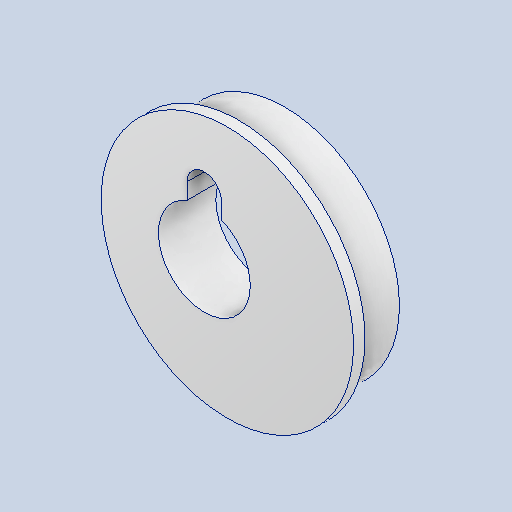
# Autodesk Inventor part: 偏心軸板
Saved by Autodesk Inventor 2024 (Build 280153000, 153)
## iProperties
Created: 2023-05-29
Part Number: 偏心軸板
Material: アルミニウム 6061
Document SubType Name: Modeling
Designer: yuta2
Density: 2.7 g/cm^3
Appearance: アルミニウム - フラット
Author: yuta2
Autodesk Inventor part; units mm, degrees
ref_plane "YZ Plane" through (0, 0, 0) normal (1, 0, 0) x (0, 1, 0)
ref_plane "XZ Plane" through (0, 0, 0) normal (0, 1, 0) x (-1, 0, 0)
ref_plane "XY Plane" through (0, 0, 0) normal (0, 0, 1) x (1, 0, 0)
sketch "スケッチ1" plane through (0, 0, 0) normal (0, 0, 1) x (1, 0, 0)
  circle A0 centre (0, 0) radius 10
  dimension "d0" = 20
  constraints: 1 centre point, 1 coincident
  measures "d0" diameter of A0
extrude "押し出し1" add sketch "スケッチ1" along normal blind 5
sketch "スケッチ2" plane through (0, 0, 5) normal (0, 0, 1) x (1, 0, 0)
  circle A0 centre (0, 0) radius 10 projected
  circle A1 centre (0, 0) radius 11
  circle A2 centre (0, 0) radius 10 projected
  dimension "d3" = 22
  constraints: 1 centre point, 1 coincident
  measures "d3" diameter of A1
extrude "押し出し2" add sketch "スケッチ2" against normal blind 1
sketch "スケッチ3" plane through (0, 0, 0) normal (0, 0, -1) x (-1, 0, 0)
  point P0 (0, 0)
  point P1 (2, 0)
  dimension "d6" = 2
  constraints: 1 horizontal alignment
  measures "d6" distance of point (0, 0) point (2, 0)
hole "穴1" at (-2, 0, 0) direction (0, 0, 1) diameter 8 end through all
sketch "スケッチ4" plane through (0, 0, 0) normal (0, 0, -1) x (-1, 0, 0)
  circle A0 centre (2, 0) radius 4 projected
  line L0 (0.5, 3.7081) -> (3.5, 3.7081)
  line L1 (3.5, 3.7081) -> (3.5, 5.1081)
  line L2 (3.5, 5.1081) -> (0.5, 5.1081)
  line L3 (0.5, 5.1081) -> (0.5, 3.7081)
  circle A1 centre (2, 5.1081) radius 1.5
  point P0 (0, 0)
  point P1 (0.5, 5.1081)
  dimension "d14" = 3
  dimension "d15" = 1.4
  constraints: 8 end point, 2 parallel, 2 point on circle, 1 horizontal, 1 midpoint, 1 perpendicular, 3 other
  measures "d14" distance of L1.end L2.end
  measures "d15" distance of L2.end L0.start
extrude "押し出し3" cut sketch "スケッチ4" against normal through all contours L0 A1 A0 | A0 A1 L1 | L3 A1 A0 | A0 A1 L0 | A1 L0 A0 | A0 A1 L2 | L2 A1 picked at (3.1128, 3.733) picked at (0.8872, 3.733) picked at (2.0995, 3.8017)
equation "\"d6\" = r"
equation "\"r\" = 2"
